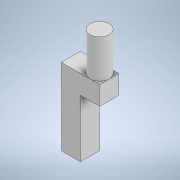
# Autodesk Inventor part: Handle
Saved by Autodesk Inventor 2022 (Build 260153000, 153)
## iProperties
Created: 2021-09-18
Part Number: Handle
Material: Generic
Document SubType Name: Modeling
Designer: marcu
Density: 1 g/cm^3
Appearance: Default
Author: marcu
Autodesk Inventor part; units mm, degrees
ref_plane "YZ Plane" through (0, 0, 0) normal (1, 0, 0) x (0, 1, 0)
ref_plane "XZ Plane" through (0, 0, 0) normal (0, 1, 0) x (-1, 0, 0)
ref_plane "XY Plane" through (0, 0, 0) normal (0, 0, 1) x (1, 0, 0)
sketch "Sketch1" plane through (0, 0, 0) normal (0, 1, 0) x (-1, 0, 0)
  line L0 (-1.5748, 1.5748) -> (1.5748, 1.5748)
  line L1 (1.5748, 1.5748) -> (1.5748, -1.5748)
  line L2 (1.5748, -1.5748) -> (-1.5748, -1.5748)
  line L3 (-1.5748, -1.5748) -> (-1.5748, 1.5748)
  line L4 (-1.5748, 1.5748) -> (1.5748, -1.5748) construction
  line L5 (1.5748, 1.5748) -> (-1.5748, -1.5748) construction
  point P0 (0, 0)
  dimension "d0" = 3.1496
  dimension "d1" = 3.1496
  constraints: 12 end point, 2 midpoint, 2 parallel, 1 horizontal, 1 perpendicular
  measures "d0" distance of L1.end L2.end
  measures "d1" distance of L0.end L1.end
extrude "Extrusion1" add sketch "Sketch1" along normal blind 6.35
sketch "Sketch2" plane through (-1.5748, 0, 1.5748) normal (0, 0, 1) x (1, 0, 0)
  line L0 (3.1496, 0) -> (0, 0) projected
  line L1 (3.1496, 0) -> (0, 0)
  line L2 (0, 0) -> (0, 12.7)
  line L3 (0, 12.7) -> (3.1496, 12.7)
  line L4 (3.1496, 12.7) -> (3.1496, 0)
  line L5 (0, 12.7) -> (6.35, 12.7)
  line L6 (6.35, 12.7) -> (6.35, 9.5504)
  line L7 (6.35, 9.5504) -> (0, 9.5504)
  line L8 (0, 9.5504) -> (0, 12.7)
  point P0 (1.5748, 0)
  point P1 (3.1496, 9.5504)
  dimension "d4" = 12.7
  dimension "d5" = 6.35
  dimension "d6" = 3.1496
  constraints: 16 end point, 4 parallel, 2 horizontal, 2 perpendicular
  measures "d4" distance of L1.end L2.end
  measures "d5" distance of L6.end L7.end
  measures "d6" distance of L5.end L6.end
extrude "Extrusion2" add sketch "Sketch2" against normal blind 3.1496
sketch "Sketch3" plane through (-1.5748, 12.7, 1.5748) normal (0, 1, 0) x (1, 0, 0)
  line L0 (0, 3.1496) -> (6.35, 3.1496) projected
  line L1 (6.35, 3.1496) -> (3.2004, 3.1496)
  line L2 (3.2004, 3.1496) -> (3.2004, 0)
  line L3 (3.2004, 0) -> (6.35, 0)
  line L4 (6.35, 0) -> (6.35, 3.1496)
  circle A0 centre (4.7752, 1.5748) radius 1.5748
  point P0 (1.5748, 1.5748)
  dimension "d9" = 3.1496
  dimension "d10" = 3.1496
  constraints: 8 end point, 2 parallel, 1 centre point, 1 horizontal, 1 perpendicular, 1 tangent
  measures "d9" distance of L3.end L2.end
  measures "d10" distance of L2.end L1.end
extrude "Extrusion3" add sketch "Sketch3" along normal blind 6.35 contours A0
body "Solid1"
